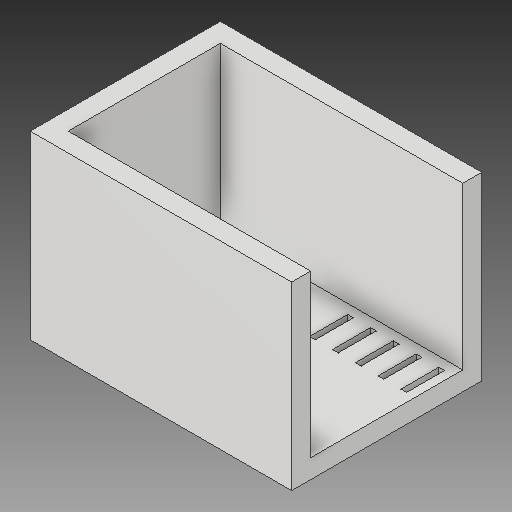
# Autodesk Inventor part: HA005
Saved by Autodesk Inventor 2017 SP1 (Build 210196100, 196)
## iProperties
Created: 2017-06-10
Part Number: HA005
Material: ABS Plastic
Document SubType Name: Modeling
Designer: Zach
Density: 1.06 g/cm^3
Appearance: CR White
Author: Zach
Autodesk Inventor part; units mm, degrees
ref_plane "YZ Plane" through (0, 0, 0) normal (1, 0, 0) x (0, 1, 0)
ref_plane "XZ Plane" through (0, 0, 0) normal (0, 1, 0) x (-1, 0, 0)
ref_plane "XY Plane" through (0, 0, 0) normal (0, 0, 1) x (1, 0, 0)
sketch "Sketch1" plane through (0, 0, 0) normal (0, 0, 1) x (1, 0, 0)
  line L0 (0, 0) -> (275, 0)
  line L1 (275, 0) -> (275, 200)
  line L2 (275, 200) -> (0, 200)
  line L3 (0, 200) -> (0, 0)
  dimension "d0" = 275
  dimension "d1" = 200
  constraints: 8 end point, 2 parallel, 1 horizontal, 1 perpendicular
  measures "d0" distance of L2.end L1.end
  measures "d1" distance of L1.end L0.end
extrude "Extrusion1" add sketch "Sketch1" along normal blind 20
sketch "Sketch3" plane through (0, 0, 20) normal (0, 0, 1) x (1, 0, 0)
  line L0 (275, 0) -> (275, 200) projected
  line L1 (0, 200) -> (275, 200)
  line L2 (275, 200) -> (275, 0)
  line L3 (275, 0) -> (0, 0)
  line L4 (0, 0) -> (0, 200)
  point P0 (0, 0)
  constraints: 8 end point, 2 parallel, 1 coincident, 1 horizontal, 1 perpendicular
extrude "Extrusion3" add sketch "Sketch3" along normal blind 80
sketch "Sketch4" plane through (0, 0, 0) normal (0, -1, 0) x (1, 0, 0)
  circle A0 centre (37.5, 50) radius 17.5
  circle A1 centre (237.5, 50) radius 17.5
  line L0 (37.5, 50) -> (237.5, 50) construction
  line L1 (0, 0) -> (0, 100) projected
  line L2 (0, 100) -> (275, 100) projected
  point P0 (0, 50)
  point P1 (137.5, 50)
  point P2 (137.5, 100)
  dimension "d10" = 35
  dimension "d11" = 35
  dimension "d12" = 200
  constraints: 3 midpoint, 2 centre point, 2 end point, 1 horizontal, 1 horizontal alignment, 1 vertical alignment
  measures "d10" diameter of A0
  measures "d11" diameter of A1
  measures "d12" distance of L0.end L0.start
extrude "Extrusion4" cut sketch "Sketch4" against normal blind 100 contours A0
sketch "Sketch5" plane through (0, 200, 0) normal (0, 1, 0) x (1, 0, 0)
  line L0 (275, 0) -> (0, 0) projected
  line L1 (0, 0) -> (0, -100) projected
  line L2 (275, -100) -> (0, -100) projected
  line L3 (275, 0) -> (275, -100) projected
  line L4 (265, -90) -> (10, -90)
  line L5 (10, -90) -> (10, -10)
  line L6 (10, -10) -> (265, -10)
  line L7 (265, -10) -> (265, -90)
  point P0 (0, 0)
  dimension "d15" = 10
  constraints: 8 end point, 3 other
  measures "d15" distance between parallel lines of L3 L7
extrude "Extrusion5" cut sketch "Sketch5" against normal blind 190 contours L4 L5 L6 L7
sketch "Sketch6" plane through (0, 0, 0) normal (-1, 0, 0) x (0, 0, 1)
  line L0 (0, 200) -> (100, 200) projected
  line L1 (0, 200) -> (0, 0) projected
  line L2 (100, 200) -> (0, 200)
  line L3 (0, 200) -> (0, 190)
  line L4 (0, 190) -> (100, 190)
  line L5 (100, 190) -> (100, 200)
  dimension "d18" = 10
  constraints: 8 end point, 2 parallel, 1 horizontal, 1 perpendicular, 1 point on line
  measures "d18" distance of L3.end L2.end
extrude "Extrusion6" cut sketch "Sketch6" against normal through all
sketch "Sketch7" plane through (0, 190, 100) normal (0, 1, 0) x (1, 0, 0)
  line L0 (275, 100) -> (275, 0) construction
  line L1 (0, 100) -> (275, 100) construction
  line L2 (0, 0) -> (0, 100) construction
  line L3 (275, 0) -> (0, 0) construction
  line L4 (265, 10) -> (265, 90) construction
  line L5 (10, 10) -> (265, 10) construction
  line L6 (10, 90) -> (10, 10) construction
  line L7 (265, 90) -> (10, 90) construction
  line L8 (270, 5) -> (270, 95) construction
  line L9 (270, 95) -> (5, 95) construction
  line L10 (5, 95) -> (5, 5) construction
  line L11 (5, 5) -> (270, 5) construction
  circle A0 centre (270, 5) radius 2.5
  circle A1 centre (270, 95) radius 2.5
  circle A2 centre (5, 95) radius 2.5
  circle A3 centre (5, 5) radius 2.5
  point P0 (0, 100)
  dimension "d21" = 5
  dimension "d22" = 5
  dimension "d23" = 5
  dimension "d24" = 5
  dimension "d25" = 5
  constraints: 8 end point, 4 centre point, 4 coincident, 3 other
  measures "d21" distance between parallel lines of L0 L8
  measures "d22" diameter of A0
  measures "d23" diameter of A1
  measures "d24" diameter of A2
  measures "d25" diameter of A3
extrude "Extrusion7" cut sketch "Sketch7" against normal blind 25
sketch "Sketch8" plane through (0, 0, 0) normal (0, -1, 0) x (1, 0, 0)
  line L0 (82, 15) -> (85, 15)
  line L1 (85, 15) -> (85, 35)
  line L2 (85, 35) -> (82, 35)
  line L3 (82, 35) -> (82, 15)
  line L4 (0, 0) -> (0, 100) projected
  line L5 (0, 0) -> (275, 0) projected
  line L6 (97, 15) -> (97, 35)
  line L7 (97, 35) -> (94, 35)
  line L8 (94, 35) -> (94, 15)
  line L9 (94, 15) -> (97, 15)
  line L10 (109, 15) -> (109, 35)
  line L11 (109, 35) -> (106, 35)
  line L12 (106, 35) -> (106, 15)
  line L13 (106, 15) -> (109, 15)
  line L14 (121, 15) -> (121, 35)
  line L15 (121, 35) -> (118, 35)
  line L16 (118, 35) -> (118, 15)
  line L17 (118, 15) -> (121, 15)
  line L18 (133, 15) -> (133, 35)
  line L19 (133, 35) -> (130, 35)
  line L20 (130, 35) -> (130, 15)
  line L21 (130, 15) -> (133, 15)
  line L22 (145, 15) -> (145, 35)
  line L23 (145, 35) -> (142, 35)
  line L24 (142, 35) -> (142, 15)
  line L25 (142, 15) -> (145, 15)
  line L26 (157, 15) -> (157, 35)
  line L27 (157, 35) -> (154, 35)
  line L28 (154, 35) -> (154, 15)
  line L29 (154, 15) -> (157, 15)
  line L30 (169, 15) -> (169, 35)
  line L31 (169, 35) -> (166, 35)
  line L32 (166, 35) -> (166, 15)
  line L33 (166, 15) -> (169, 15)
  line L34 (181, 15) -> (181, 35)
  line L35 (181, 35) -> (178, 35)
  line L36 (178, 35) -> (178, 15)
  line L37 (178, 15) -> (181, 15)
  line L38 (193, 15) -> (193, 35)
  line L39 (193, 35) -> (190, 35)
  line L40 (190, 35) -> (190, 15)
  line L41 (190, 15) -> (193, 15)
  line L42 (205, 15) -> (205, 35)
  line L43 (205, 35) -> (202, 35)
  line L44 (202, 35) -> (202, 15)
  line L45 (202, 15) -> (205, 15)
  line L46 (217, 15) -> (217, 35)
  line L47 (217, 35) -> (214, 35)
  line L48 (214, 35) -> (214, 15)
  line L49 (214, 15) -> (217, 15)
  line L50 (229, 15) -> (229, 35)
  line L51 (229, 35) -> (226, 35)
  line L52 (226, 35) -> (226, 15)
  line L53 (226, 15) -> (229, 15)
  line L54 (241, 15) -> (241, 35)
  line L55 (241, 35) -> (238, 35)
  line L56 (238, 35) -> (238, 15)
  line L57 (238, 15) -> (241, 15)
  dimension "d28" = 3
  dimension "d29" = 20
  dimension "d30" = 82
  dimension "d31" = 15
  dimension "d34" = 12
  constraints: 112 end point, 2 horizontal, 2 parallel, 1 perpendicular, 104 other
  measures "d28" distance of L2.end L1.end
  measures "d29" distance of L1.end L0.end
  measures "d30" distance between parallel lines of L4 L3
  measures "d31" distance between parallel lines of L5 L0
  measures "d34" distance of L0.end L6.start
extrude "Extrusion8" cut sketch "Sketch8" against normal through all
sketch "Sketch2" plane through (275, 0, 100) normal (1, 0, 0) x (0, 0, -1)
  circle A0 centre (70, 125) radius 3
  line L0 (100, 0) -> (0, 0) projected
  line L1 (100, 0) -> (100, 190) projected
  dimension "d4" = 6
  dimension "d45" = 125
  dimension "d46" = 30
  constraints: 1 centre point
  measures "d4" diameter of A0
  measures "d45" distance from line of A0.centre L0
  measures "d46" distance from line of L1 A0.centre
extrude "Extrusion2" cut sketch "Sketch2" against normal through all
sketch "Sketch10" plane through (0, 190, 100) normal (0, 1, 0) x (1, 0, 0)
  line L0 (275, 100) -> (275, 0) projected
  line L1 (0, 0) -> (275, 0) projected
  line L2 (275, 100) -> (137.5, 100)
  line L3 (137.5, 100) -> (137.5, 0)
  line L4 (137.5, 0) -> (275, 0)
  line L5 (275, 0) -> (275, 100)
  point P0 (0, 100)
  constraints: 8 end point, 2 parallel, 1 horizontal, 1 midpoint, 1 perpendicular
extrude "Extrusion10" cut sketch "Sketch10" against normal through all
sketch "Sketch11" plane through (10, 10, 90) normal (1, 0, 0) x (0, 0, -1)
  circle A0 centre (60, 123.75) radius 1.5
  circle A1 centre (60, 106.25) radius 1.5
  circle A2 centre (60, 115) radius 3 projected
  line L0 (60, 106.25) -> (60, 123.75) construction
  point P0 (90, -10)
  dimension "d49" = 3
  dimension "d50" = 3
  dimension "d51" = 17.5
  constraints: 2 centre point, 2 end point, 1 coincident, 1 midpoint, 1 vertical
  measures "d49" diameter of A0
  measures "d50" diameter of A1
  measures "d51" distance of L0.start L0.end
extrude "Extrusion11" cut sketch "Sketch11" against normal through all contours A0 | A1
sketch "Sketch12" plane through (10, 10, 90) normal (1, 0, 0) x (0, 0, -1)
  circle A0 centre (60, 115) radius 3 projected
  circle A1 centre (60, 115) radius 5
  point P0 (90, -10)
  dimension "d54" = 10
  constraints: 1 centre point, 1 coincident
  measures "d54" diameter of A1
extrude "Extrusion12" cut sketch "Sketch12" against normal blind 8
sketch "Sketch13" plane through (10, 10, 90) normal (1, 0, 0) x (0, 0, -1)
  circle A0 centre (60, 115) radius 5 projected
  circle A1 centre (60, 115) radius 3 projected
  circle A2 centre (60, 115) radius 14
  point P0 (90, -10)
  dimension "d57" = 28
  constraints: 1 centre point, 1 coincident
  measures "d57" diameter of A2
extrude "Extrusion13" cut sketch "Sketch13" against normal blind 5 contours A2
sketch "Sketch14" plane through (0, 0, 100) normal (0, 0, 1) x (1, 0, 0)
  line L0 (0, 190) -> (0, 0) projected
  line L1 (137.5, 10) -> (137.5, 190) projected
  line L2 (0, 190) -> (137.5, 190)
  line L3 (137.5, 190) -> (137.5, 95)
  line L4 (137.5, 95) -> (0, 95)
  line L5 (0, 95) -> (0, 190)
  dimension "d60" = 95
  constraints: 8 end point, 2 parallel, 1 horizontal, 1 perpendicular, 1 point on line
  measures "d60" distance of L2.end L3.end
extrude "Extrusion14" cut sketch "Sketch14" against normal through all
body "Solid1"
